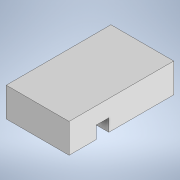
# Autodesk Inventor part: FP Rear Hood
Saved by Autodesk Inventor 2020 (Build 240168000, 168)
## iProperties
Created: 2021-04-14
Part Number: FP Rear Hood
Material: Generic
Document SubType Name: Modeling
Designer: austi
Density: 1 g/cm^3
Appearance: Default
Author: austi
Autodesk Inventor part; units mm, degrees
ref_plane "YZ Plane" through (0, 0, 0) normal (1, 0, 0) x (0, 1, 0)
ref_plane "XZ Plane" through (0, 0, 0) normal (0, 1, 0) x (-1, 0, 0)
ref_plane "XY Plane" through (0, 0, 0) normal (0, 0, 1) x (1, 0, 0)
sketch "Sketch1" plane through (0, 0, 0) normal (0, 1, 0) x (-1, 0, 0)
  line L0 (9.8, 0) -> (-9.8, 0) projected
  line L1 (0, -35) -> (0, 35) projected
  line L2 (7, 25) -> (-7, 25)
  line L3 (-7, -25) -> (7, -25)
  line L4 (7, -25) -> (7, 25)
  line L5 (-7, 12) -> (-1, 12)
  line L6 (-1, 12) -> (-1, 6)
  line L7 (-1, 6) -> (-7, 6)
  line L8 (-7, 25) -> (-7, 12)
  line L9 (-7, 6) -> (-7, -25)
  point P0 (0, 0)
  point P1 (7, 0)
  point P2 (0, 25)
  dimension "d0" = 14
  dimension "d1" = 50
  dimension "d2" = 6
  dimension "d3" = 6
  dimension "d4" = 13
  constraints: 16 end point, 5 perpendicular, 4 parallel, 2 horizontal, 2 midpoint, 1 horizontal alignment, 1 vertical alignment, 1 other
  measures "d0" distance of L3.end L3.start
  measures "d1" distance of L3.start L2.end
  measures "d2" distance of L5.start L5.end
  measures "d3" distance of L5.end L6.end
  measures "d4" distance of L5.start L2.end
extrude "Extrusion1" add sketch "Sketch1" along normal blind 30
body "Solid1"
